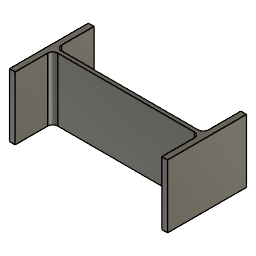
H-250×125×6×9 (Autodesk Fusion 360 design; units mm, degrees)
Autodesk Fusion 360 part; units mm, degrees
sketch "スケッチ1" plane through (0, 0, 0) normal (0, 0, 1) x (1, 0, 0)
  line L0 (0, 62.5) -> (0, -62.5)
  line L1 (9, 11) -> (9, 62.5)
  line L2 (241, 62.5) -> (241, 11)
  line L3 (250, -62.5) -> (250, 62.5)
  line L4 (233, 3) -> (17, 3)
  line L5 (17, -3) -> (233, -3)
  line L6 (9, -62.5) -> (9, -11)
  line L7 (0, -62.5) -> (9, -62.5)
  line L8 (241, -11) -> (241, -62.5)
  line L9 (241, -62.5) -> (250, -62.5)
  line L10 (9, 62.5) -> (0, 62.5)
  line L11 (250, 62.5) -> (241, 62.5)
  arc A0 (9, 11) -> (17, 3) centre (17, 11) ccw
  arc A1 (17, -3) -> (9, -11) centre (17, -11) ccw
  arc A2 (241, -11) -> (233, -3) centre (233, -11) ccw
  arc A3 (233, 3) -> (241, 11) centre (233, 11) ccw
extrude "押し出し1" add sketch "スケッチ1" along normal blind 100
